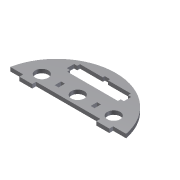
# Autodesk Inventor part: OpenROV_Dev_EChassis_Plug_Mount
Saved by Autodesk Inventor 2012 (Build 160160000, 160)
## iProperties
Created: 2012-08-07
Part Number: OpenROV_Dev_EChassis_Plug_Mount
Material: Default
Document SubType Name: Modeling
Designer: user
Density: 1 g/cm^3
Author: user
Autodesk Inventor part; units mm, degrees
ref_plane "YZ Plane" through (0, 0, 0) normal (1, 0, 0) x (0, 1, 0)
ref_plane "XZ Plane" through (0, 0, 0) normal (0, 1, 0) x (-1, 0, 0)
ref_plane "XY Plane" through (0, 0, 0) normal (0, 0, 1) x (1, 0, 0)
sketch "Sketch1" plane through (0, 0, 0) normal (0, 0, 1) x (1, 0, 0)
  arc A0 (45.111, 9) -> (-45.111, 9) centre (0, 0) ccw
  line L0 (35, 9) -> (35, 6)
  line L1 (35, 6) -> (25, 6)
  line L2 (25, 6) -> (25, 9)
  line L3 (-25, 9) -> (-25, 6)
  line L4 (-25, 6) -> (-35, 6)
  line L5 (-35, 6) -> (-35, 9)
  line L6 (-45.111, 9) -> (-35, 9)
  line L7 (-25, 9) -> (25, 9)
  line L8 (35, 9) -> (45.111, 9)
  line L9 (-22.2, 35.8) -> (-22.2, 30.2)
  line L10 (-22.2, 30.2) -> (-19.75, 30.2)
  line L11 (-19.75, 30.2) -> (-19.75, 28)
  line L12 (19.75, 28) -> (19.75, 30.2)
  line L13 (19.75, 30.2) -> (22.2, 30.2)
  line L14 (22.2, 30.2) -> (22.2, 35.8)
  line L15 (22.2, 35.8) -> (19.75, 35.8)
  line L16 (19.75, 35.8) -> (19.75, 38)
  line L17 (19.75, 38) -> (2, 38)
  line L18 (2, 38) -> (2, 39.6)
  line L19 (2, 39.6) -> (-2, 39.6)
  line L20 (-2, 39.6) -> (-2, 38)
  line L21 (-2, 38) -> (-19.75, 38)
  line L22 (-19.75, 38) -> (-19.75, 35.8)
  line L23 (-19.75, 35.8) -> (-22.2, 35.8)
  line L24 (-19.75, 28) -> (19.75, 28)
  line L25 (-15.5, 19) -> (-12.5, 19)
  line L26 (-12.5, 19) -> (-12.5, 14)
  line L27 (-12.5, 14) -> (-15.5, 14)
  line L28 (-15.5, 14) -> (-15.5, 19)
  line L29 (12.5, 19) -> (15.5, 19)
  line L30 (15.5, 19) -> (15.5, 14)
  line L31 (15.5, 14) -> (12.5, 14)
  line L32 (12.5, 14) -> (12.5, 19)
  circle A1 centre (0, 16.5) radius 5
  circle A2 centre (-28, 16.5) radius 5
  circle A3 centre (28, 16.5) radius 5
  dimension "d7" = 46
  dimension "d8" = 50
  dimension "d9" = 10
  dimension "d10" = 10
  dimension "d12" = 5.6
  dimension "d13" = 2.2
  dimension "d14" = 4
  dimension "d15" = 39.5
  dimension "d17" = 5.6
  dimension "d18" = 2.2
  dimension "d22" = 17.75
  dimension "d23" = 44.4
  dimension "d24" = 39.5
  dimension "d25" = 2.2
  dimension "d26" = 2.2
  dimension "d27" = 2.45
  dimension "d28" = 2.45
  dimension "d29" = 11.6
  dimension "d30" = 22.2
  dimension "d31" = 28
  dimension "d34" = 5
  dimension "d35" = 3
  dimension "d36" = 5
  dimension "d37" = 3
  dimension "d38" = 5
  dimension "d39" = 5
  dimension "d40" = 25
  dimension "d41" = 12.5
  dimension "d44" = 10
  dimension "d45" = 10
  dimension "d46" = 10
  dimension "d47" = 12.5
  dimension "d48" = 12.5
  dimension "d49" = 12.5
  constraints: 66 end point, 20 parallel, 9 perpendicular, 4 centre point, 2 horizontal, 2 point on circle, 1 coincident, 1 collinear
  measures "d7" radius of A0
  measures "d8" distance between parallel lines of L2 L3
  measures "d9" distance between parallel lines of L3 L5
  measures "d10" distance between parallel lines of L0 L2
  measures "d12" distance between parallel lines of L13 L15
  measures "d13" distance between parallel lines of L17 L15
  measures "d14" distance between parallel lines of L20 L18
  measures "d15" distance between parallel lines of L22 L16
  measures "d17" distance between parallel lines of L10 L23
  measures "d18" distance between parallel lines of L21 L23
  measures "d22" distance between parallel lines of L22 L20
  measures "d23" distance between parallel lines of L14 L9
  measures "d24" distance between parallel lines of L12 L11
  measures "d25" distance between parallel lines of L24 L13
  measures "d26" distance between parallel lines of L24 L10
  measures "d27" distance between parallel lines of L9 L22
  measures "d28" distance between parallel lines of L11 L9
  measures "d29" distance between parallel lines of L24 L19
  measures "d30" distance from line of point (0, 0) L9
  measures "d31" distance from line of point (0, 0) L24
  measures "d34" distance between parallel lines of L27 L25
  measures "d35" distance between parallel lines of L26 L28
  measures "d36" distance between parallel lines of L31 L29
  measures "d37" distance between parallel lines of L30 L32
  measures "d38" distance between parallel lines of L7 L31
  measures "d39" distance between parallel lines of L7 L27
  measures "d40" distance between parallel lines of L32 L26
  measures "d41" distance from line of point (0, 0) L26
  measures "d44" diameter of A1
  measures "d45" diameter of A2
  measures "d46" diameter of A3
  measures "d47" distance from line of L32 A1.centre
  measures "d48" distance from line of L28 A2.centre
  measures "d49" distance from line of L30 A3.centre
extrude "Extrusion3" add sketch "Sketch1" along normal blind 3
body "Solid3"
